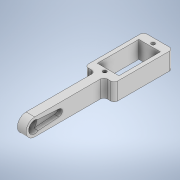
# Autodesk Inventor part: link3
Saved by Autodesk Inventor 2020.2 (Build 242310000, 310)
## iProperties
Created: 2026-05-18
Part Number: link3
Material: Generic
Document SubType Name: Modeling
Designer: explorer
Density: 1 g/cm^3
Appearance: Default
Author: explorer
Autodesk Inventor part; units mm, degrees
ref_plane "YZ Plane" through (0, 0, 0) normal (1, 0, 0) x (0, 1, 0)
ref_plane "XZ Plane" through (0, 0, 0) normal (0, 1, 0) x (-1, 0, 0)
ref_plane "XY Plane" through (0, 0, 0) normal (0, 0, 1) x (1, 0, 0)
sketch "Sketch2" plane through (0, 0, 0) normal (1, 0, 0) x (0, 1, 0)
  circle A0 centre (0, 0) radius 3.5
  line L0 (5, 0) -> (5, -40)
  line L1 (5, -40) -> (-5, -40)
  line L2 (-5, -40) -> (-5, 0)
  line L3 (-5, 0) -> (5, 0) construction
  arc A1 (5, 0) -> (-5, 0) centre (0, 0) ccw
  line L4 (0, 0) -> (5, 0) construction
  line L5 (0, 0) -> (0, 5) construction
  line L6 (0, 0) -> (-5, 0) construction
  point P0 (-5, 0)
  dimension "d1" = 7
  dimension "d2" = 5
  dimension "d3" = 90
  dimension "d4" = 180
  dimension "d11" = 40
  constraints: 14 end point, 3 coincident, 2 centre point, 2 parallel, 2 perpendicular, 2 point on circle, 1 midpoint, 1 tangent, 1 vertical
  measures "d1" diameter of A0
  measures "d2" radius of A1
  measures "d3" angle of L4 L5
  measures "d4" angle of L4 L6
  measures "d11" distance of L2.start L2.end
extrude "Extrusion1" add sketch "Sketch2" along normal mid plane 5
sketch "Sketch4" plane through (-2.5, 5, 0) normal (0, 1, 0) x (1, 0, 0)
  line L0 (2.5, 89.8) -> (2.5, -20.8) projected
  line L1 (-9.4, 0) -> (14.4, 0) projected
  line L2 (-6, 74) -> (11, 74)
  line L3 (11, 74) -> (11, 40)
  line L4 (11, 40) -> (-6, 40)
  line L5 (-6, 40) -> (-6, 74)
  line L6 (-6, 57) -> (11, 57) construction
  line L7 (-3.75, 69) -> (8.75, 69)
  line L8 (8.75, 69) -> (8.75, 45)
  line L9 (8.75, 45) -> (-3.75, 45)
  line L10 (-3.75, 45) -> (-3.75, 69)
  line L11 (-3.75, 69) -> (8.75, 45) construction
  line L12 (8.75, 69) -> (-3.75, 45) construction
  line L13 (5, 40) -> (0, 40) projected
  line L14 (2.5, 71) -> (2.5, 43) construction
  circle A0 centre (2.5, 71) radius 1.05
  circle A1 centre (2.5, 43) radius 1.05
  point P0 (2.5, 0)
  point P1 (2.5, 57)
  point P2 (2.5, 40)
  point P3 (2.5, 57)
  dimension "d18" = 34
  dimension "d19" = 17
  dimension "d20" = 12.5
  dimension "d21" = 24
  dimension "d22" = 2.1
  dimension "d23" = 28
  constraints: 24 end point, 9 midpoint, 4 parallel, 2 centre point, 2 coincident, 2 horizontal, 2 perpendicular, 1 equal radius, 1 point on line, 1 vertical
  measures "d18" distance of L2.end L3.end
  measures "d19" distance of L2.start L2.end
  measures "d20" distance of L7.start L7.end
  measures "d21" distance of L7.end L8.end
  measures "d22" diameter of A0
  measures "d23" distance of L14.start L14.end
extrude "Extrusion3" add sketch "Sketch4" against normal up to surface (10 mm away) contours L2 L3 L4 L0 A1 L9 L8 L7 A0 | L0 A0 L7 L10 L9 A1 L4 L5 L2
sketch "Sketch5" plane through (2.5, 0, 0) normal (1, 0, 0) x (0, 0, -1)
  circle A0 centre (0, 0) radius 3
  arc A1 (14, -2) -> (14, 2) centre (14, 0) ccw
  line L0 (14, 0) -> (14, 2) construction
  line L1 (14, 0) -> (16, 0) construction
  line L2 (14, 0) -> (14, -2) construction
  line L3 (0, 11.9) -> (0, -11.9)
  line L4 (14, 2) -> (0, 3)
  line L5 (14, -2) -> (0, -3)
  point P0 (0.4264, -2.9695)
  point P1 (0.4264, 2.9695)
  dimension "d27" = 6
  dimension "d28" = 90
  dimension "d29" = 180
  dimension "d30" = 14
  dimension "d31" = 2
  constraints: 12 end point, 4 point on circle, 2 centre point, 2 point on line, 1 coincident, 1 horizontal, 1 perpendicular, 1 vertical
  measures "d27" diameter of A0
  measures "d28" angle of L1 L0
  measures "d29" angle of L0 L2
  measures "d30" distance of L0.start point (0, 0)
  measures "d31" radius of A1
fillet "Fillet1" radius 2 6 edges at (2.5, 0, -40) (8.5, 0, -40) (8.5, 0, -74) (-8.5, 0, -74) (-8.5, 0, -40) (-2.5, 0, -40)
extrude "Extrusion4" cut sketch "Sketch5" against normal blind 2.5
body "Solid1"
